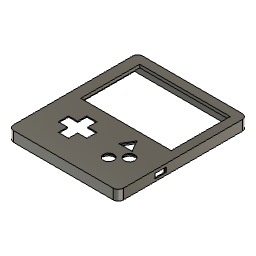
FINAL BMO Enclosure ECE 196 (Autodesk Fusion 360 design; units mm, degrees)
Autodesk Fusion 360 part; units mm, degrees
(part 1 of 2)
sketch "Sketch1" plane through (0, 0, 0) normal (0, 0, 1) x (1, 0, 0)
  line L0 (-50.4372, 47.8193) -> (49.5628, 47.8193)
  line L1 (49.5628, 47.8193) -> (49.5628, -63.1807)
  line L2 (49.5628, -63.1807) -> (-50.4372, -63.1807)
  line L3 (-50.4372, -63.1807) -> (-50.4372, 47.8193)
  line L4 (-18.6372, -27.5802) -> (-23.0372, -27.5802)
  line L5 (-23.0372, -27.5802) -> (-23.0372, -24.2802)
  line L6 (-23.0372, -24.2802) -> (-18.6372, -24.2802)
  line L7 (-18.6372, -24.2802) -> (-18.6372, -27.5802)
  line L8 (17.6628, -24.0807) -> (22.0628, -24.0807)
  line L9 (22.0628, -24.0807) -> (22.0628, -27.3807)
  line L10 (22.0628, -27.3807) -> (17.6628, -27.3807)
  line L11 (17.6628, -27.3807) -> (17.6628, -24.0807)
  line L12 (17.8378, -44.4057) -> (22.2378, -44.4057)
  line L13 (22.2378, -44.4057) -> (22.2378, -47.7057)
  line L14 (22.2378, -47.7057) -> (17.8378, -47.7057)
  line L15 (17.8378, -47.7057) -> (17.8378, -44.4057)
  line L16 (27.9628, -34.1807) -> (32.3628, -34.1807)
  line L17 (32.3628, -34.1807) -> (32.3628, -37.4807)
  line L18 (32.3628, -37.4807) -> (27.9628, -37.4807)
  line L19 (27.9628, -37.4807) -> (27.9628, -34.1807)
  line L20 (-33.0372, -34.1807) -> (-28.6372, -34.1807)
  line L21 (-28.6372, -34.1807) -> (-28.6372, -37.4807)
  line L22 (-28.6372, -37.4807) -> (-33.0372, -37.4807)
  line L23 (-33.0372, -37.4807) -> (-33.0372, -34.1807)
  line L24 (-13.0372, -34.1807) -> (-8.6372, -34.1807)
  line L25 (-8.6372, -34.1807) -> (-8.6372, -37.4807)
  line L26 (-8.6372, -37.4807) -> (-13.0372, -37.4807)
  line L27 (-13.0372, -37.4807) -> (-13.0372, -34.1807)
  line L28 (-23.4439, -44.4057) -> (-19.0439, -44.4057)
  line L29 (-19.0439, -44.4057) -> (-19.0439, -47.7057)
  line L30 (-19.0439, -47.7057) -> (-23.4439, -47.7057)
  line L31 (-23.4439, -47.7057) -> (-23.4439, -44.4057)
  dimension "d1" = 100
  dimension "d2" = 111
  dimension "d3" = 4.4
  dimension "d4" = 3.3
  dimension "d5" = 4.4
  dimension "d6" = 3.3
  dimension "d7" = 4.4
  dimension "d8" = 3.3
  dimension "d9" = 4.4
  dimension "d10" = 3.3
  dimension "d11" = 4.4
  dimension "d12" = 3.3
  dimension "d13" = 4.4
  dimension "d14" = 3.3
  dimension "d15" = 4.4
  dimension "d16" = 3.3
  dimension "d17" = 17.4
  dimension "d21" = 25.7
  dimension "d22" = 25.7
  dimension "d23" = 15.475
  dimension "d24" = 15.475
  dimension "d25" = 25.7
  dimension "d26" = 27.5
  dimension "d27" = 17.2
  dimension "d28" = 15.6
  dimension "d29" = 8.656
  dimension "d30" = 8.656
  dimension "d31" = 8.656
  dimension "d32" = 35.8
  dimension "d33" = 27.325
  constraint horizontal L0
  constraint vertical L1
  constraint horizontal L2
  constraint vertical L3
  constraint horizontal L4
  constraint vertical L5
  constraint horizontal L6
  constraint vertical L7
  constraint horizontal L8
  constraint vertical L9
  constraint horizontal L10
  constraint vertical L11
  constraint horizontal L12
  constraint vertical L13
  constraint horizontal L14
  constraint vertical L15
  constraint horizontal L16
  constraint vertical L17
  constraint horizontal L18
  constraint vertical L19
  constraint horizontal L20
  constraint vertical L21
  constraint horizontal L22
  constraint vertical L23
  constraint horizontal L24
  constraint vertical L25
  constraint horizontal L26
  constraint vertical L27
  constraint horizontal L28
  constraint vertical L29
  constraint horizontal L30
  constraint vertical L31
  measures "d1" distance of L0.start L0.end
  measures "d2" distance of L0.end L1.end
  measures "d3" distance of L4.start L4.end
  measures "d4" distance of L4.end L5.end
  measures "d5" distance of L28.start L28.end
  measures "d6" distance of L28.end L29.end
  measures "d7" distance of L24.start L24.end
  measures "d8" distance of L24.end L25.end
  measures "d9" distance of L20.start L20.end
  measures "d10" distance of L20.end L21.end
  measures "d11" distance of L8.start L8.end
  measures "d12" distance of L8.end L9.end
  measures "d13" distance of L16.start L16.end
  measures "d14" distance of L16.end L17.end
  measures "d15" distance of L12.start L12.end
  measures "d16" distance of L12.start L14.end
  measures "d17" distance of L3 L23
  measures "d21" distance of L2 L22
  measures "d22" distance of L2 L26
  measures "d23" distance of L2 L30
  measures "d24" distance of L2 L14
  measures "d25" distance of L2 L18
  measures "d26" distance of L1 L9
  measures "d27" distance of L1 L17
  measures "d28" distance of L21 L27
  measures "d29" distance of L4.end L20.end
  measures "d30" distance of L4.start L24.start
  measures "d31" distance of L21.end L28.start
  measures "d32" distance of L2 L10
  measures "d33" distance of L1 L13
sketch "top enclosure" plane through (0, 0, 0) normal (0, 0, 1) x (1, 0, 0)
  circle A0 centre (30.5628, -36.1807) radius 5.15
  line L0 (20.0628, -18.1807) -> (13.3583, -29.4363)
  line L1 (13.3583, -29.4363) -> (26.3583, -29.4363)
  line L2 (26.3583, -29.4363) -> (20.0628, -18.1807)
  circle A1 centre (20.0628, -46.1807) radius 5.15
  line L3 (-25.9372, -21.6807) -> (-15.9372, -21.6807)
  line L4 (-15.9372, -21.6807) -> (-15.9372, -30.6807)
  line L5 (-15.9372, -30.6807) -> (-6.9372, -30.6807)
  line L6 (-6.9372, -30.6807) -> (-6.9372, -40.6807)
  line L7 (-6.9372, -40.6807) -> (-15.9372, -40.6807)
  line L8 (-15.9372, -40.6807) -> (-15.9372, -49.6807)
  line L9 (-15.9372, -49.6807) -> (-25.9372, -49.6807)
  line L10 (-25.9372, -49.6807) -> (-25.9372, -40.6807)
  line L11 (-25.9372, -40.6807) -> (-34.9372, -40.6807)
  line L12 (-34.9372, -40.6807) -> (-34.9372, -30.6807)
  line L13 (-34.9372, -30.6807) -> (-25.9372, -30.6807)
  line L14 (-25.9372, -30.6807) -> (-25.9372, -21.6807)
  line L15 (-54.4372, 56.8193) -> (53.5628, 56.8193)
  line L16 (53.5628, 56.8193) -> (53.5628, -70.1807)
  line L17 (53.5628, -70.1807) -> (-54.4372, -70.1807)
  line L18 (-54.4372, -70.1807) -> (-54.4372, 56.8193)
  line L19 (-50.4372, -63.1807) -> (-50.4372, 47.8193)
  line L20 (49.5628, -63.1807) -> (-50.4372, -63.1807)
  line L21 (49.5628, 47.8193) -> (49.5628, -63.1807)
  line L22 (-50.4372, 47.8193) -> (49.5628, 47.8193)
  line L23 (-43.9372, 48.3193) -> (45.0628, 48.3193)
  line L24 (45.0628, 48.3193) -> (45.0628, -9.6807)
  line L25 (45.0628, -9.6807) -> (-43.9372, -9.6807)
  line L26 (-43.9372, -9.6807) -> (-43.9372, 48.3193)
  line L27 (-23.0372, -24.2802) -> (-18.6372, -24.2802)
  line L28 (-50.4372, -63.1807) -> (49.5628, -63.1807)
  line L29 (49.5628, -63.1807) -> (49.5628, 49.8193)
  line L30 (49.5628, 49.8193) -> (-50.4372, 49.8193)
  line L31 (-50.4372, 49.8193) -> (-50.4372, -63.1807)
  line L32 (44.9628, -13.6807) -> (49.5628, -13.6807)
  line L33 (49.5628, -13.6807) -> (49.5628, -23.1807)
  line L34 (49.5628, -23.1807) -> (44.9628, -23.1807)
  line L35 (44.9628, -23.1807) -> (44.9628, -13.6807)
  line L36 (-50.4372, -5.1807) -> (-36.8011, -5.1807)
  line L37 (-36.8011, -5.1807) -> (-36.8011, -27.1807)
  line L38 (-36.8011, -27.1807) -> (-50.4372, -27.1807)
  line L39 (-50.4372, -27.1807) -> (-50.4372, -5.1807)
  dimension "d34" = 60
  dimension "d35" = 10.3
  dimension "d36" = 10.3
  dimension "d37" = 10
  dimension "d38" = 10
  dimension "d39" = 10
  dimension "d40" = 10
  dimension "d41" = 9
  dimension "d42" = 9
  dimension "d43" = 9
  dimension "d44" = 9
  dimension "d45" = 9
  dimension "d46" = 9
  dimension "d47" = 13
  dimension "d49" = 11.2555
  dimension "d50" = 4
  dimension "d51" = 7
  dimension "d52" = 4
  dimension "d54" = 89
  dimension "d55" = 58
  dimension "d56" = 6.5
  dimension "d59" = 14.5995
  dimension "d60" = 45
  dimension "d61" = 27
  dimension "d62" = 17
  dimension "d63" = 13.5
  dimension "d64" = 15.5
  dimension "d65" = 19
  dimension "d66" = 29.5
  dimension "d68" = 113
  dimension "d69" = 100
  dimension "d72" = 40
  dimension "d73" = 9.5
  dimension "d74" = 4.6
  dimension "d75" = 36
  dimension "d77" = 22
  dimension "d230" = 7
  constraint horizontal L1
  constraint horizontal L3
  constraint perpendicular L3 L4
  constraint perpendicular L4 L5
  constraint perpendicular L5 L6
  constraint perpendicular L6 L7
  constraint perpendicular L7 L8
  constraint perpendicular L8 L9
  constraint perpendicular L9 L10
  constraint perpendicular L10 L11
  constraint perpendicular L11 L12
  constraint perpendicular L12 L13
  constraint perpendicular L3 L14
  constraint horizontal L15
  constraint vertical L16
  constraint horizontal L17
  constraint vertical L18
  constraint horizontal L23
  constraint vertical L24
  constraint horizontal L25
  constraint vertical L26
  constraint horizontal L28
  constraint vertical L29
  constraint horizontal L30
  constraint vertical L31
  constraint coincident L19.start L20.end
  constraint horizontal L32
  constraint vertical L33
  constraint horizontal L34
  constraint vertical L35
  constraint coincident L21 L33.end
  constraint horizontal L36
  constraint vertical L37
  constraint horizontal L38
  constraint vertical L39
  constraint coincident L19 L36.start
  measures "d34" angle of L0 L2
  measures "d35" diameter of A1
  measures "d36" diameter of A0
  measures "d37" distance of L3.start L3.end
  measures "d38" distance of L8.end L9.end
  measures "d39" distance of L5.end L6.end
  measures "d40" distance of L11.end L12.end
  measures "d41" distance of L3.start L13.end
  measures "d42" distance of L3.end L4.end
  measures "d43" distance of L4.end L5.end
  measures "d44" distance of L6.end L7.end
  measures "d45" distance of L9.end L10.end
  measures "d46" distance of L12.end L13.end
  measures "d47" distance of L0.end L1.end
  measures "d49" distance of L0.start L1
  measures "d50" distance of L18 L19
  measures "d51" distance of L17 L20
  measures "d52" distance of L16 L21
  measures "d54" distance of L23.start L23.end
  measures "d55" distance of L23.end L24.end
  measures "d56" distance of L19 L26
  measures "d59" distance of L25 L27
  measures "d60" distance of L0.start L20
  measures "d61" distance of A0.centre L20
  measures "d62" distance of A1.centre L20
  measures "d63" distance of L9 L20
  measures "d64" distance of L12 L19
  measures "d65" distance of A0.centre L21
  measures "d66" distance of L0.start L21
  measures "d68" distance of L19.start L30.end
  measures "d69" distance of L19.start L20.start
  measures "d72" distance of L20 L34
  measures "d73" distance of L32 L34
  measures "d74" distance of L33 L35
  measures "d75" distance of L28 L38
  measures "d77" distance of L36.end L37.end
  measures "d230" distance of L15 L30
extrude "Extrude6" add sketch "top enclosure" along normal blind 10 contours L15 L16 L17 L18 makes body 1
extrude "Extrude7" add sketch "top enclosure" along normal blind 3 contours L19 L20 L21 L22 L24 L25 L28 L29 L31 L32 L34 L35 L37 L38 | L19 L25 L26 L31 L36 L37 L38 L39 | L19 L22 L26 L31 L36 | L21 L29 L32 L33 L34 L35 | L22 L23 L24 L26 L29 L30 L31 bodies 1
sketch "Sketch3" plane through (53.5628, 0, 0) normal (1, 0, 0) x (0, 1, 0)
  line L0 (-70.1807, 0) -> (56.8193, 0)
  line L1 (56.8193, 0) -> (56.8193, 10)
  line L2 (56.8193, 10) -> (-70.1807, 10)
  line L3 (-70.1807, 10) -> (-70.1807, 0)
  line L4 (-34.1807, 7.5) -> (-23.1807, 7.5)
  line L5 (-23.1807, 7.5) -> (-23.1807, 3)
  line L6 (-23.1807, 3) -> (-34.1807, 3)
  line L7 (-34.1807, 3) -> (-34.1807, 7.5)
  line L8 (56.8193, 0) -> (-70.1807, 0)
  line L9 (-63.1807, 3) -> (-63.1807, 10)
  dimension "d92" = 3
  dimension "d93" = 11
  dimension "d94" = 4.5
  dimension "d212" = 40
  constraint horizontal L4
  constraint vertical L5
  constraint horizontal L6
  constraint vertical L7
  measures "d92" distance of L6 L8
  measures "d93" distance of L4.start L4.end
  measures "d94" distance of L4.end L5.end
  measures "d212" distance of L5 L9
extrude "Extrude8" cut sketch "Sketch3" against normal blind 10 contours L4 L5 L6 L7 bodies 1
sketch "Sketch4" plane through (49.5628, 0, 0) normal (-1, 0, 0) x (0, -1, 0)
  line L0 (23.1807, 3) -> (23.1807, 7.5)
  line L1 (23.1807, 7.5) -> (34.1807, 7.5)
  line L2 (34.1807, 7.5) -> (34.1807, 3)
  line L3 (34.1807, 3) -> (63.1807, 3)
  line L4 (63.1807, 3) -> (63.1807, 10)
  line L5 (63.1807, 10) -> (-49.8193, 10)
  line L6 (-49.8193, 10) -> (-49.8193, 3)
  line L7 (-49.8193, 3) -> (23.1807, 3)
  line L8 (21.9307, 3) -> (33.9307, 3)
  line L9 (33.9307, 3) -> (33.9307, 13)
  line L10 (33.9307, 13) -> (21.9307, 13)
  line L11 (21.9307, 13) -> (21.9307, 3)
  line L12 (23.1807, 7.5) -> (23.1807, 3)
  dimension "d97" = 12
  dimension "d98" = 10
  dimension "d99" = 1.25
  constraint horizontal L8
  constraint vertical L9
  constraint horizontal L10
  constraint vertical L11
  constraint coincident L7 L8.start
  measures "d97" distance of L9.end L10.end
  measures "d98" distance of L8.end L9.end
  measures "d99" distance of L11 L12
sketch "Sketch5" plane through (-54.4372, 0, 0) normal (-1, 0, 0) x (0, -1, 0)
  line L0 (-56.8193, 0) -> (70.1807, 0)
  line L1 (70.1807, 0) -> (70.1807, 10)
  line L2 (70.1807, 10) -> (-56.8193, 10)
  line L3 (-56.8193, 10) -> (-56.8193, 0)
  line L4 (8.1807, 7.5) -> (26.1807, 7.5)
  line L5 (26.1807, 7.5) -> (26.1807, 3)
  line L6 (26.1807, 3) -> (8.1807, 3)
  line L7 (8.1807, 3) -> (8.1807, 7.5)
  line L8 (63.1807, 3) -> (63.1807, 10)
  dimension "d103" = 18
  dimension "d104" = 3
  dimension "d105" = 4.5
  dimension "d174" = 55
  constraint horizontal L4
  constraint vertical L5
  constraint horizontal L6
  constraint vertical L7
  measures "d103" distance of L4.start L4.end
  measures "d104" distance of L0 L6
  measures "d105" distance of L4.end L5.end
  measures "d174" distance of L7 L8
sketch "Sketch6" plane through (-50.4372, 0, 0) normal (1, 0, 0) x (0, 1, 0)
  line L0 (49.8193, 3) -> (49.8193, 10)
  line L1 (49.8193, 10) -> (-63.1807, 10)
  line L2 (-63.1807, 10) -> (-63.1807, 3)
  line L3 (-63.1807, 3) -> (49.8193, 3)
  line L4 (-28.6807, 3) -> (-6.6807, 3)
  line L5 (-6.6807, 3) -> (-6.6807, 13)
  line L6 (-6.6807, 13) -> (-28.6807, 13)
  line L7 (-28.6807, 13) -> (-28.6807, 3)
  dimension "d111" = 22
  dimension "d112" = 10
  constraint horizontal L4
  constraint vertical L5
  constraint horizontal L6
  constraint vertical L7
  constraint coincident L3 L4.start
  measures "d111" distance of L5.end L6.end
  measures "d112" distance of L4.start L6.end
extrude "Extrude11" cut sketch "Sketch6" against normal blind 3 contours L1 L3 L4 L5 L7 | L1 L5 L6 L7 bodies 1
sketch "Sketch7" plane through (0, 0, 10) normal (0, 0, 1) x (-1, 0, 0)
  line L0 (50.4372, 28.6807) -> (53.4372, 28.6807)
  line L1 (53.4372, 28.6807) -> (53.4372, 6.6807)
  line L2 (53.4372, 6.6807) -> (50.4372, 6.6807)
  line L3 (50.4372, 6.6807) -> (50.4372, -49.8193)
  line L4 (50.4372, -49.8193) -> (-49.5628, -49.8193)
  line L5 (-49.5628, -49.8193) -> (-49.5628, 63.1807)
  line L6 (-49.5628, 63.1807) -> (50.4372, 63.1807)
  line L7 (50.4372, 63.1807) -> (50.4372, 28.6807)
  line L8 (54.4372, 70.1807) -> (-53.5628, 70.1807)
  line L9 (-53.5628, 70.1807) -> (-53.5628, -56.8193)
  line L10 (-53.5628, -56.8193) -> (54.4372, -56.8193)
  line L11 (54.4372, -56.8193) -> (54.4372, 70.1807)
  line L12 (54.4372, -56.8193) -> (-53.5628, -56.8193)
  line L13 (-53.5628, -56.8193) -> (-53.5628, 70.1807)
  line L14 (-53.5628, 70.1807) -> (54.4372, 70.1807)
  line L15 (54.4372, 70.1807) -> (54.4372, -56.8193)
  line L16 (50.4372, -49.8193) -> (-49.5628, -49.8193)
  line L17 (-49.5628, -49.8193) -> (-49.5628, 63.1807)
  line L18 (-49.5628, 63.1807) -> (50.4372, 63.1807)
  line L19 (50.4372, 63.1807) -> (50.4372, -49.8193)
  constraint horizontal L12
  constraint vertical L13
  constraint horizontal L14
  constraint vertical L15
  constraint coincident L8.end L9.start
  constraint coincident L10.end L11.start
  constraint horizontal L16
  constraint vertical L17
  constraint horizontal L18
  constraint vertical L19
  constraint coincident L5.end L6.start
  constraint coincident L3.end L4.start
extrude "Extrude12" add sketch "Sketch7" along normal blind 18.5 separate body contours L3 L4 L5 L6 L7 L16 L17 L18 L19 | L0 L1 L2 L19 | L8 L9 L10 L11 L12 L13 L14 L15 makes body 2
extrude "Extrude13" cut sketch "Sketch7" along normal blind 16 contours L3 L4 L5 L6 L7 L16 L17 L18 L19 bodies 2
sketch "Sketch9" plane through (53.5628, 0, 0) normal (1, 0, 0) x (0, 1, 0)
  line L0 (-70.1807, 10) -> (56.8193, 10)
  line L1 (56.8193, 10) -> (56.8193, 28.5)
  line L2 (56.8193, 28.5) -> (-70.1807, 28.5)
  line L3 (-70.1807, 28.5) -> (-70.1807, 10)
  line L4 (11.7578, 25.9206) -> (-35.8078, 25.9206) construction
  line L5 (-35.8078, 25.9206) -> (-35.8078, 11.4906) construction
  line L6 (-35.8078, 11.4906) -> (11.7578, 11.4906) construction
  line L7 (11.7578, 11.4906) -> (11.7578, 25.9206) construction
  dimension "d118" = 13
sketch "Sketch11" plane through (0, 0, 26) normal (0, 0, -1) x (1, 0, 0)
  line L0 (49.5628, 63.1807) -> (-50.4372, 63.1807)
  line L1 (-50.4372, 63.1807) -> (-50.4372, -49.8193)
  line L2 (-50.4372, -49.8193) -> (49.5628, -49.8193)
  line L3 (49.5628, -49.8193) -> (49.5628, 63.1807)
  line L4 (24.494, -23.0885) -> (41.494, -23.0885)
  line L5 (41.494, -23.0885) -> (41.494, 2.9115)
  line L6 (41.494, 2.9115) -> (24.494, 2.9115)
  line L7 (24.494, 2.9115) -> (24.494, -23.0885)
  ellipse E0 centre (32.994, -10.0885) end of major axis (32.994, 0) minor radius 7.0905
  line L8 (32.994, -20.177) -> (32.994, 0) construction
  line L9 (40.0845, -10.0885) -> (25.9034, -10.0885) construction
  dimension "d129" = 26
  dimension "d130" = 17
  constraint horizontal L4
  constraint vertical L5
  constraint horizontal L6
  constraint vertical L7
  constraint coincident E0 L8.start
  constraint coincident E0 L8.end
  constraint coincident E0 L9.start
  constraint coincident E0 L9.end
  constraint perpendicular L4 L8
  measures "d129" distance of L4.start L6.end
  measures "d130" distance of L5.end L6.end
sketch "Sketch12" plane through (0, 0, 3) normal (0, 0, 1) x (-1, 0, 0)
  line L0 (50.4372, 28.6807) -> (50.4372, 63.1807)
  line L1 (50.4372, 63.1807) -> (-49.5628, 63.1807)
  line L2 (-49.5628, 63.1807) -> (-49.5628, 34.1807)
  line L3 (-49.5628, 34.1807) -> (-53.5628, 34.1807)
  line L4 (-53.5628, 34.1807) -> (-53.5628, 23.1807)
  line L5 (-53.5628, 23.1807) -> (-49.5628, 23.1807)
  line L6 (-49.5628, 23.1807) -> (-49.5628, -49.8193)
  line L7 (-49.5628, -49.8193) -> (50.4372, -49.8193)
  line L8 (50.4372, -49.8193) -> (50.4372, 6.6807)
  line L9 (50.4372, 6.6807) -> (53.4372, 6.6807)
  line L10 (53.4372, 6.6807) -> (53.4372, 28.6807)
  line L11 (-45.0628, -48.3193) -> (-45.0628, 9.6807)
  line L12 (-45.0628, 9.6807) -> (43.9372, 9.6807)
  line L13 (43.9372, 9.6807) -> (43.9372, -48.3193)
  line L14 (43.9372, -48.3193) -> (-45.0628, -48.3193)
  circle A0 centre (-30.5628, 36.1807) radius 5.15
  line L15 (-20.0628, 18.1807) -> (-26.3583, 29.4363)
  line L16 (-26.3583, 29.4363) -> (-13.3583, 29.4363)
  line L17 (-13.3583, 29.4363) -> (-20.0628, 18.1807)
  circle A1 centre (-20.0628, 46.1807) radius 5.15
  line L18 (34.9372, 30.6807) -> (25.9372, 30.6807)
  line L19 (25.9372, 30.6807) -> (25.9372, 21.6807)
  line L20 (25.9372, 21.6807) -> (15.9372, 21.6807)
  line L21 (15.9372, 21.6807) -> (15.9372, 30.6807)
  line L22 (15.9372, 30.6807) -> (6.9372, 30.6807)
  line L23 (6.9372, 30.6807) -> (6.9372, 40.6807)
  line L24 (6.9372, 40.6807) -> (15.9372, 40.6807)
  line L25 (15.9372, 40.6807) -> (15.9372, 49.6807)
  line L26 (15.9372, 49.6807) -> (25.9372, 49.6807)
  line L27 (25.9372, 49.6807) -> (25.9372, 40.6807)
  line L28 (25.9372, 40.6807) -> (34.9372, 40.6807)
  line L29 (34.9372, 40.6807) -> (34.9372, 30.6807)
  line L30 (15.9372, 30.6807) -> (6.9372, 30.6807)
  line L31 (6.9372, 30.6807) -> (6.9372, 40.6807)
  line L32 (15.9372, 40.6807) -> (15.9372, 49.6807)
  line L33 (15.9372, 49.6807) -> (25.9372, 49.6807)
  line L34 (25.9372, 49.6807) -> (25.9372, 40.6807)
  line L35 (34.9372, 40.6807) -> (34.9372, 30.6807)
  line L36 (34.9372, 30.6807) -> (25.9372, 30.6807)
  line L37 (25.9372, 21.6807) -> (15.9372, 21.6807)
  line L38 (15.9372, 21.6807) -> (15.9372, 30.6807)
  line L39 (25.9372, 30.6807) -> (25.9372, 21.6807)
  line L40 (-28.0634, 30.4363) -> (-11.5986, 30.4363)
  line L41 (-11.5986, 30.4363) -> (-20.0901, 16.1809)
  line L42 (-20.0901, 16.1809) -> (-28.0634, 30.4363)
  circle A2 centre (-30.5628, 36.1807) radius 6.15
  circle A3 centre (-20.0628, 46.1807) radius 6.15
  line L43 (4.9372, 28.6807) -> (4.9372, 42.6807)
  line L44 (4.9372, 42.6807) -> (13.9372, 42.6807)
  line L45 (13.9372, 42.6807) -> (13.9372, 51.6807)
  line L46 (13.9372, 51.6807) -> (27.9372, 51.6807)
  line L47 (27.9372, 51.6807) -> (27.9372, 42.6807)
  line L48 (27.9372, 42.6807) -> (36.9372, 42.6807)
  line L49 (36.9372, 42.6807) -> (36.9372, 28.6807)
  line L50 (36.9372, 28.6807) -> (27.9372, 28.6807)
  line L51 (27.9372, 28.6807) -> (27.9372, 19.6807)
  line L52 (27.9372, 19.6807) -> (13.9372, 19.6807)
  line L53 (13.9372, 19.6807) -> (13.9372, 28.6807)
  line L54 (13.9372, 28.6807) -> (4.9372, 28.6807)
  line L55 (53.4372, 28.6807) -> (50.4372, 28.6807)
  line L56 (-13.965, 45.3815) -> (-10, 45.3815)
  line L57 (-10, 45.3815) -> (-10, 48)
  line L58 (-10, 48) -> (-14.188, 48)
  line L59 (-36.6796, 36.8191) -> (-40.3994, 36.8191)
  line L60 (-40.3994, 36.8191) -> (-40.3994, 34)
  line L61 (-40.3994, 34) -> (-36.3132, 34)
  line L62 (-13.965, 45.3815) -> (-14.188, 48)
  line L63 (-36.3132, 34) -> (-36.6796, 36.8191)
  dimension "d145" = -1
  dimension "d146" = 1
  dimension "d147" = 1
  dimension "d148" = -2
  constraint coincident A3 L56.start
  constraint horizontal L56
  constraint perpendicular L56 L57
  constraint coincident A3 L58.end
  constraint perpendicular L57 L58
  constraint coincident A2 L59.start
  constraint parallel L12 L59
  constraint perpendicular L12 L60
  constraint coincident A2 L61.end
  constraint perpendicular L60 L61
extrude "Extrude20" cut sketch "Sketch12" against normal blind 2 contours L43 L44 L45 L46 L47 L48 L49 L50 L51 L52 L53 L54 bodies 1
extrude "Extrude21" cut sketch "Sketch12" against normal blind 2 contours L40 L41 L42 | A2 L63 | A2 L63 | A2 L59 L60 L61 | A3 L62 | A3 L56 L57 L58 | A3 L62 bodies 1
sketch "Sketch13" plane through (49.5628, 0, 0) normal (-1, 0, 0) x (0, -1, 0)
  line L0 (23.1807, 3) -> (23.1807, 7.5)
  line L1 (23.1807, 7.5) -> (34.1807, 7.5)
  line L2 (34.1807, 7.5) -> (34.1807, 3)
  line L3 (34.1807, 3) -> (63.1807, 3)
  line L4 (63.1807, 3) -> (63.1807, 10)
  line L5 (63.1807, 10) -> (-49.8193, 10)
  line L6 (-49.8193, 10) -> (-49.8193, 3)
  line L7 (-49.8193, 3) -> (23.1807, 3)
  line L8 (21.1807, 3) -> (36.1807, 3)
  line L9 (36.1807, 3) -> (36.1807, 11.5)
  line L10 (36.1807, 11.5) -> (21.1807, 11.5)
  line L11 (21.1807, 11.5) -> (21.1807, 3)
  dimension "d154" = 2
  dimension "d155" = 2
  dimension "d156" = 4
  constraint horizontal L8
  constraint vertical L9
  constraint horizontal L10
  constraint vertical L11
  constraint coincident L7 L8.start
  measures "d154" distance of L0 L11
  measures "d155" distance of L2 L9
  measures "d156" distance of L1 L10
extrude "Extrude22" cut sketch "Sketch13" against normal blind 3 contours L0 L1 L2 L3 L5 L7 L8 L9 L11 bodies 1
fillet "Fillet1" radius 5 1 edges at (-54.4372, 56.8193, 19.25) on bodies 2
fillet "Fillet2" radius 5 1 edges at (-54.4372, 56.8193, 5) on bodies 1
fillet "Fillet3" radius 5 2 edges at (-54.4372, -70.1807, 5) (-54.4372, -70.1807, 19.25) on bodies 1 2
fillet "Fillet4" radius 5 2 edges at (53.5628, 56.8193, 5) (53.5628, 56.8193, 19.25) on bodies 1 2
fillet "Fillet5" radius 5 2 edges at (53.5628, -70.1807, 5) (53.5628, -70.1807, 19.25) on bodies 1 2
sketch "Sketch14" plane through (0, 0, 1) normal (0, 0, 1) x (-1, 0, 0)
  line L0 (34.9372, 30.6807) -> (25.9372, 30.6807)
  line L1 (25.9372, 30.6807) -> (25.9372, 21.6807)
  line L2 (25.9372, 21.6807) -> (15.9372, 21.6807)
  line L3 (15.9372, 21.6807) -> (15.9372, 30.6807)
  line L4 (15.9372, 30.6807) -> (6.9372, 30.6807)
  line L5 (6.9372, 30.6807) -> (6.9372, 40.6807)
  line L6 (6.9372, 40.6807) -> (15.9372, 40.6807)
  line L7 (15.9372, 40.6807) -> (15.9372, 49.6807)
  line L8 (15.9372, 49.6807) -> (25.9372, 49.6807)
  line L9 (25.9372, 49.6807) -> (25.9372, 40.6807)
  line L10 (25.9372, 40.6807) -> (34.9372, 40.6807)
  line L11 (34.9372, 40.6807) -> (34.9372, 30.6807)
  line L12 (13.9372, 28.6807) -> (13.9372, 19.6807)
  line L13 (13.9372, 19.6807) -> (27.9372, 19.6807)
  line L14 (27.9372, 19.6807) -> (27.9372, 28.6807)
  line L15 (27.9372, 28.6807) -> (36.9372, 28.6807)
  line L16 (36.9372, 28.6807) -> (36.9372, 42.6807)
  line L17 (36.9372, 42.6807) -> (27.9372, 42.6807)
  line L18 (27.9372, 42.6807) -> (27.9372, 51.6807)
  line L19 (27.9372, 51.6807) -> (13.9372, 51.6807)
  line L20 (13.9372, 51.6807) -> (13.9372, 42.6807)
  line L21 (13.9372, 42.6807) -> (4.9372, 42.6807)
  line L22 (4.9372, 42.6807) -> (4.9372, 28.6807)
  line L23 (4.9372, 28.6807) -> (13.9372, 28.6807)
  line L24 (14.7372, 20.4807) -> (27.1372, 20.4807)
  line L25 (27.1372, 20.4807) -> (27.1372, 29.4807)
  line L26 (27.1372, 29.4807) -> (36.1372, 29.4807)
  line L27 (36.1372, 29.4807) -> (36.1372, 41.8807)
  line L28 (36.1372, 41.8807) -> (27.1372, 41.8807)
  line L29 (27.1372, 41.8807) -> (27.1372, 50.8807)
  line L30 (27.1372, 50.8807) -> (14.7372, 50.8807)
  line L31 (14.7372, 50.8807) -> (14.7372, 41.8807)
  line L32 (14.7372, 41.8807) -> (5.7372, 41.8807)
  line L33 (5.7372, 41.8807) -> (5.7372, 29.4807)
  line L34 (5.7372, 29.4807) -> (14.7372, 29.4807)
  line L35 (14.7372, 29.4807) -> (14.7372, 20.4807)
  dimension "d175" = -0.8
sketch "Sketch15" plane through (0, 0, 1) normal (0, 0, 1) x (-1, 0, 0)
  line L0 (-26.3583, 29.4363) -> (-13.3583, 29.4363)
  line L1 (-13.3583, 29.4363) -> (-20.0628, 18.1807)
  line L2 (-20.0628, 18.1807) -> (-26.3583, 29.4363)
  line L3 (-20.0901, 16.1809) -> (-11.5986, 30.4363)
  line L4 (-11.5986, 30.4363) -> (-28.0634, 30.4363)
  line L5 (-28.0634, 30.4363) -> (-20.0901, 16.1809)
  line L6 (-12.3025, 30.0363) -> (-27.3813, 30.0363)
  line L7 (-27.3813, 30.0363) -> (-20.0791, 16.9808)
  line L8 (-20.0791, 16.9808) -> (-12.3025, 30.0363)
  dimension "d176" = -0.4
sketch "Sketch16" plane through (0, 0, 1) normal (0, 0, 1) x (-1, 0, 0)
  circle A0 centre (-30.5628, 36.1807) radius 5.15
  circle A1 centre (-30.5628, 36.1807) radius 5.75
  line L0 (-40.3994, 34) -> (-36.3132, 34)
  arc A2 (-36.3132, 34) -> (-36.6796, 36.8191) centre (-30.5628, 36.1807) ccw
  line L1 (-36.6796, 36.8191) -> (-40.3994, 36.8191)
  line L2 (-40.3994, 36.8191) -> (-40.3994, 34)
  line L3 (-36.0013, 34.3137) -> (-40, 34.3137)
  line L4 (-40, 34.3137) -> (-40, 36.5)
  line L5 (-40, 36.5) -> (-36.3039, 36.5)
  constraint coincident A1 L3.start
  constraint horizontal L3
  constraint perpendicular L3 L4
  constraint coincident A1 L5.end
  constraint perpendicular L4 L5
sketch "Sketch17" plane through (0, 0, 1) normal (0, 0, 1) x (-1, 0, 0)
  circle A0 centre (-20.0628, 46.1807) radius 5.15
  circle A1 centre (-20.0628, 46.1807) radius 5.75
  line L0 (-10, 48) -> (-14.188, 48)
  arc A2 (-14.188, 48) -> (-13.965, 45.3815) centre (-20.0628, 46.1807) ccw
  line L1 (-13.965, 45.3815) -> (-10, 45.3815)
  line L2 (-10, 45.3815) -> (-10, 48)
  line L3 (-14.332, 45.7107) -> (-10.2595, 45.7107)
  line L4 (-10.2595, 45.7107) -> (-10.2595, 47.6884)
  line L5 (-10.2595, 47.6884) -> (-14.514, 47.6884)
  constraint coincident A1 L3.start
  constraint parallel L1 L3
  constraint perpendicular L3 L4
  constraint coincident A1 L5.end
  constraint perpendicular L4 L5
extrude "Extrude23" add sketch "Sketch14" sketch "Sketch15" sketch "Sketch16" sketch "Sketch17" along normal up to surface separate body contours L0 L1 L2 L3 L4 L5 L6 L7 L8 L9 L10 L11 | L24 L25 L26 L27 L28 L29 L30 L31 L32 L33 L34 L35 of sketch 2 contours L0 L1 L2 | L6 L7 L8 of sketch 3 contours A0 | A1 | A1 L3 L4 L5 of sketch 4 contours A0 | A1 | A1 L3 L4 L5 end surface through (0, 0, 10) normal (0, 0, 1) offset -4.6 makes body 3 at (35.053, -32.589, 3.9333) makes body 4 at (19.921, -25.6845, 1) makes body 5 at (-23.0039, -37.7474, 1) makes body 6 at (24.8522, -42.9988, 3.9333)
sketch "Sketch22" plane through (0, 0, 1) normal (0, 0, -1) x (1, 0, 0)
  line L0 (12.3025, 30.0363) -> (20.0791, 16.9808)
  line L1 (20.0791, 16.9808) -> (27.3813, 30.0363)
  line L2 (27.3813, 30.0363) -> (12.3025, 30.0363)
  line L3 (26.0172, 29.2363) -> (13.7102, 29.2363)
  line L4 (13.7102, 29.2363) -> (20.0573, 18.5807)
  line L5 (20.0573, 18.5807) -> (26.0172, 29.2363)
  dimension "d187" = -0.8
sketch "Sketch23" plane through (0, 0, 1) normal (0, 0, -1) x (1, 0, 0)
  circle A0 centre (30.5628, 36.1807) radius 4.85
  arc A1 (36.3039, 36.5) -> (36.0013, 34.3137) centre (30.5628, 36.1807) ccw
  line L0 (36.0013, 34.3137) -> (40, 34.3137)
  line L1 (40, 34.3137) -> (40, 36.5)
  line L2 (40, 36.5) -> (36.3039, 36.5)
  line L3 (12.3025, 30.0363) -> (20.0791, 16.9808)
  line L4 (20.0791, 16.9808) -> (27.3813, 30.0363)
  line L5 (27.3813, 30.0363) -> (12.3025, 30.0363)
  line L6 (14.514, 47.6884) -> (10.2595, 47.6884)
  line L7 (10.2595, 47.6884) -> (10.2595, 45.7107)
  line L8 (10.2595, 45.7107) -> (14.332, 45.7107)
  arc A2 (14.332, 45.7107) -> (14.514, 47.6884) centre (20.0628, 46.1807) ccw
  line L9 (-14.7372, 20.4807) -> (-14.7372, 29.4807)
  line L10 (-14.7372, 29.4807) -> (-5.7372, 29.4807)
  line L11 (-5.7372, 29.4807) -> (-5.7372, 41.8807)
  line L12 (-5.7372, 41.8807) -> (-14.7372, 41.8807)
  line L13 (-14.7372, 41.8807) -> (-14.7372, 50.8807)
  line L14 (-14.7372, 50.8807) -> (-27.1372, 50.8807)
  line L15 (-27.1372, 50.8807) -> (-27.1372, 41.8807)
  line L16 (-27.1372, 41.8807) -> (-36.1372, 41.8807)
  line L17 (-36.1372, 41.8807) -> (-36.1372, 29.4807)
  line L18 (-36.1372, 29.4807) -> (-27.1372, 29.4807)
  line L19 (-27.1372, 29.4807) -> (-27.1372, 20.4807)
  line L20 (-27.1372, 20.4807) -> (-14.7372, 20.4807)
  constraint concentric A0 A1
sketch "Sketch24" plane through (0, 0, 1) normal (0, 0, -1) x (1, 0, 0)
  line L0 (-14.7372, 20.4807) -> (-14.7372, 29.4807)
  line L1 (-14.7372, 29.4807) -> (-5.7372, 29.4807)
  line L2 (-5.7372, 29.4807) -> (-5.7372, 41.8807)
  line L3 (-5.7372, 41.8807) -> (-14.7372, 41.8807)
  line L4 (-14.7372, 41.8807) -> (-14.7372, 50.8807)
  line L5 (-14.7372, 50.8807) -> (-27.1372, 50.8807)
  line L6 (-27.1372, 50.8807) -> (-27.1372, 41.8807)
  line L7 (-27.1372, 41.8807) -> (-36.1372, 41.8807)
  line L8 (-36.1372, 41.8807) -> (-36.1372, 29.4807)
  line L9 (-36.1372, 29.4807) -> (-27.1372, 29.4807)
  line L10 (-27.1372, 29.4807) -> (-27.1372, 20.4807)
  line L11 (-27.1372, 20.4807) -> (-14.7372, 20.4807)
  line L12 (-16.2372, 30.9807) -> (-7.2372, 30.9807)
  line L13 (-7.2372, 30.9807) -> (-7.2372, 40.3807)
  line L14 (-7.2372, 40.3807) -> (-16.2372, 40.3807)
  line L15 (-16.2372, 40.3807) -> (-16.2372, 49.3807)
  line L16 (-16.2372, 49.3807) -> (-25.6372, 49.3807)
  line L17 (-25.6372, 49.3807) -> (-25.6372, 40.3807)
  line L18 (-25.6372, 40.3807) -> (-34.6372, 40.3807)
  line L19 (-34.6372, 40.3807) -> (-34.6372, 30.9807)
  line L20 (-34.6372, 30.9807) -> (-25.6372, 30.9807)
  line L21 (-25.6372, 30.9807) -> (-25.6372, 21.9807)
  line L22 (-25.6372, 21.9807) -> (-16.2372, 21.9807)
  line L23 (-16.2372, 21.9807) -> (-16.2372, 30.9807)
  dimension "d189" = -1.5
sketch "Sketch25" plane through (0, 0, 1) normal (0, 0, -1) x (1, 0, 0)
  circle A0 centre (30.5628, 36.1807) radius 4.85
  arc A1 (36.3039, 36.5) -> (36.0013, 34.3137) centre (30.5628, 36.1807) ccw
  line L0 (36.0013, 34.3137) -> (40, 34.3137)
  line L1 (40, 34.3137) -> (40, 36.5)
  line L2 (40, 36.5) -> (36.3039, 36.5)
  line L3 (12.3025, 30.0363) -> (20.0791, 16.9808)
  line L4 (20.0791, 16.9808) -> (27.3813, 30.0363)
  line L5 (27.3813, 30.0363) -> (12.3025, 30.0363)
  line L6 (14.514, 47.6884) -> (10.2595, 47.6884)
  line L7 (10.2595, 47.6884) -> (10.2595, 45.7107)
  line L8 (10.2595, 45.7107) -> (14.332, 45.7107)
  arc A2 (14.332, 45.7107) -> (14.514, 47.6884) centre (20.0628, 46.1807) ccw
  line L9 (-14.7372, 20.4807) -> (-14.7372, 29.4807)
  line L10 (-14.7372, 29.4807) -> (-5.7372, 29.4807)
  line L11 (-5.7372, 29.4807) -> (-5.7372, 41.8807)
  line L12 (-5.7372, 41.8807) -> (-14.7372, 41.8807)
  line L13 (-14.7372, 41.8807) -> (-14.7372, 50.8807)
  line L14 (-14.7372, 50.8807) -> (-27.1372, 50.8807)
  line L15 (-27.1372, 50.8807) -> (-27.1372, 41.8807)
  line L16 (-27.1372, 41.8807) -> (-36.1372, 41.8807)
  line L17 (-36.1372, 41.8807) -> (-36.1372, 29.4807)
  line L18 (-36.1372, 29.4807) -> (-27.1372, 29.4807)
  line L19 (-27.1372, 29.4807) -> (-27.1372, 20.4807)
  line L20 (-27.1372, 20.4807) -> (-14.7372, 20.4807)
  circle A3 centre (20.0628, 46.1807) radius 5.1598
  circle A4 centre (20.0628, 46.1807) radius 4.8598
  dimension "d207" = -0.3
  constraint concentric A0 A1
  constraint concentric A2 A3
extrude "Extrude25" add sketch "Sketch23" sketch "Sketch22" sketch "Sketch25" sketch "Sketch24" along normal blind 2.5 contours A0 of sketch 2 contours L3 L4 L5 of sketch 3 contours A0 of sketch 4 contours L12 L13 L14 L15 L16 L17 L18 L19 L20 L21 L22 L23 bodies 3 5 4
sketch "Sketch26" plane through (0, 0, -1.5) normal (0, 0, -1) x (1, 0, 0)
  line L0 (-16.2372, 21.9807) -> (-16.2372, 30.9807)
  line L1 (-16.2372, 30.9807) -> (-7.2372, 30.9807)
  line L2 (-7.2372, 30.9807) -> (-7.2372, 40.3807)
  line L3 (-7.2372, 40.3807) -> (-16.2372, 40.3807)
  line L4 (-16.2372, 40.3807) -> (-16.2372, 49.3807)
  line L5 (-16.2372, 49.3807) -> (-25.6372, 49.3807)
  line L6 (-25.6372, 49.3807) -> (-25.6372, 40.3807)
  line L7 (-25.6372, 40.3807) -> (-34.6372, 40.3807)
  line L8 (-34.6372, 40.3807) -> (-34.6372, 30.9807)
  line L9 (-34.6372, 30.9807) -> (-25.6372, 30.9807)
  line L10 (-25.6372, 30.9807) -> (-25.6372, 21.9807)
  line L11 (-25.6372, 21.9807) -> (-16.2372, 21.9807)
  circle A0 centre (-20.9372, 35.6807) radius 3
  dimension "d193" = 6
  measures "d193" diameter of A0
extrude "Extrude26" cut sketch "Sketch26" against normal blind 0.3 contours A0 bodies 5
fillet "Fillet6" radius 0.3 1 edges at (-23.7342, -36.7656, -1.5) on bodies 5
sketch "Sketch27" plane through (0, 0, -1.5) normal (0, 0, -1) x (1, 0, 0)
  line L0 (20.0573, 18.5807) -> (26.0172, 29.2363)
  line L1 (26.0172, 29.2363) -> (13.7102, 29.2363)
  line L2 (13.7102, 29.2363) -> (20.0573, 18.5807)
  line L3 (21, 28) -> (19, 28) construction
  line L4 (19, 28) -> (19, 23) construction
  line L5 (19, 23) -> (21, 23) construction
  line L6 (21, 23) -> (21, 28) construction
  line L7 (32.948, 39.073) -> (28.0236, 39.0916) construction
  line L8 (28.0236, 39.0916) -> (28.0006, 33.0191) construction
  line L9 (28.0006, 33.0191) -> (32.925, 33.0005) construction
  line L10 (32.925, 33.0005) -> (32.948, 39.073) construction
  line L11 (22.1916, 49.0811) -> (17.5135, 49.0529) construction
  line L12 (17.5135, 49.0529) -> (17.5465, 43.5713) construction
  line L13 (17.5465, 43.5713) -> (22.2246, 43.5995) construction
  line L14 (22.2246, 43.5995) -> (22.1916, 49.0811) construction
  dimension "d198" = 5
  dimension "d199" = 5
  dimension "d200" = 5
  text T0 "S" font "Arial" height 5 align centre middle in box 2 x 5 at (21, 28) x (-1, 0) y (0, -1) spacing 1 kerned
  text T1 "D" font "Arial" height 5 align centre middle in box 4.9245 x 6.0725 at (32.948, 39.073) x (-0.999993, 0.003785) y (-0.003785, -0.999993) spacing 1 kerned
  text T2 "B" font "Arial" height 5 align centre middle in box 4.6781 x 5.4817 at (22.1916, 49.0811) x (-0.999982, -0.006022) y (0.006022, -0.999982) spacing 1 kerned
extrude "Extrude28" cut sketch "Sketch27" against normal blind 0.5 text T1 T2 T0 bodies 3 4
extrude "Extrude29" cut sketch "Sketch27" against normal blind 0.6 text T0 bodies 4
extrude "Extrude30" add sketch "Sketch25" along normal blind 2.5 contours A4 bodies 6
extrude "Extrude31" cut sketch "Sketch27" against normal blind 0.5 text T2 bodies 6
sketch "Sketch29" plane through (-54.4372, 0, 0) normal (-1, 0, 0) x (0, -1, 0)
  line L0 (28.6079, 8.2636) -> (6.6079, 8.2636)
  line L1 (6.6079, 8.2636) -> (6.6079, 14.2636)
  line L2 (6.6079, 14.2636) -> (28.6079, 14.2636)
  line L3 (28.6079, 14.2636) -> (28.6079, 8.2636)
  dimension "d213" = 6
  dimension "d214" = 22
  constraint horizontal L0
  constraint vertical L1
  constraint horizontal L2
  constraint vertical L3
  measures "d213" distance of L0.start L2.end
  measures "d214" distance of L0.start L0.end
extrude "Extrude32" cut sketch "Sketch29" against normal blind 6 bodies 1 2
sketch "Sketch30" plane through (49.5628, 0, 0) normal (-1, 0, 0) x (0, -1, 0)
  line L0 (-49.8193, 10) -> (63.1807, 10)
  line L1 (63.1807, 10) -> (63.1807, 26)
  line L2 (63.1807, 26) -> (-49.8193, 26)
  line L3 (-49.8193, 26) -> (-49.8193, 10)
  line L4 (-23.7308, 10.6685) -> (-38.7308, 10.6685)
  line L5 (-23.8198, 25.7685) -> (-38.8198, 25.7685)
  arc A0 (-23.7308, 10.6685) -> (-23.8198, 25.7685) centre (-25.1353, 18.2105) ccw
  arc A1 (-38.8198, 25.7685) -> (-38.7308, 10.6685) centre (-37.6054, 18.2254) ccw
  circle A2 centre (-31.599, 12.6391) radius 1.25
  circle A3 centre (-31.4598, 17.937) radius 1.25
  circle A4 centre (-26.9413, 15.1675) radius 1.25
  circle A5 centre (-26.8021, 20.4654) radius 1.25
  circle A6 centre (-31.3206, 23.235) radius 1.25
  circle A7 centre (-35.9784, 20.7066) radius 1.25
  circle A8 centre (-36.1176, 15.4086) radius 1.25
  dimension "d217" = 15.1
  dimension "d218" = 15
  dimension "d219" = 15
  dimension "d220" = 7.6717
  dimension "d221" = 7.6402
  dimension "d224" = 2.5
  dimension "d225" = 2.5
  dimension "d227" = 360
  constraint horizontal L4
  constraint parallel L2 L5
  measures "d217" distance of L4 L5
  measures "d218" distance of L4.start L4.end
  measures "d219" distance of L5.start L5.end
  measures "d220" radius of A0
  measures "d221" radius of A1
  measures "d224" diameter of A2
  measures "d225" diameter of A3
extrude "Extrude33" cut sketch "Sketch30" against normal blind 3.3 contours L4 L5 A0 A1 | A2 | A3 | A4 | A5 | A6 | A7 | A8 bodies 2
extrude "Extrude34" cut sketch "Sketch30" against normal blind 5 contours A2 | A3 | A4 | A5 | A6 | A7 | A8 bodies 2
sketch "Sketch31" plane through (0, 0, 10) normal (0, 0, -1) x (1, 0, 0)
  line L0 (-50.4372, 6.6079) -> (-54.4372, 6.6079)
  line L1 (-54.4372, 6.6079) -> (-54.4372, -51.8193)
  arc A0 (-54.4372, -51.8193) -> (-49.4372, -56.8193) centre (-49.4372, -51.8193) ccw
  line L2 (-49.4372, -56.8193) -> (48.5628, -56.8193)
  arc A1 (48.5628, -56.8193) -> (53.5628, -51.8193) centre (48.5628, -51.8193) ccw
  line L3 (53.5628, -51.8193) -> (53.5628, 65.1807)
  arc A2 (53.5628, 65.1807) -> (48.5628, 70.1807) centre (48.5628, 65.1807) ccw
  line L4 (48.5628, 70.1807) -> (-49.4372, 70.1807)
  arc A3 (-49.4372, 70.1807) -> (-54.4372, 65.1807) centre (-49.4372, 65.1807) ccw
  line L5 (-54.4372, 65.1807) -> (-54.4372, 28.6079)
  line L6 (-54.4372, 28.6079) -> (-50.4372, 28.6079)
  line L7 (-50.4372, 28.6079) -> (-50.4372, 63.1807)
  line L8 (-50.4372, 63.1807) -> (49.5628, 63.1807)
  line L9 (49.5628, 63.1807) -> (49.5628, -49.8193)
  line L10 (49.5628, -49.8193) -> (-50.4372, -49.8193)
  line L11 (-50.4372, -49.8193) -> (-50.4372, 6.6079)
  circle A4 centre (-36.2346, 66.4664) radius 2.725
  circle A5 centre (37.4116, 66.6526) radius 2.725
  circle A6 centre (-36.7046, -53.3293) radius 2.725
  circle A7 centre (35.1958, -53.3905) radius 2.725
  circle A8 centre (-36.2346, 66.4664) radius 1.5
  circle A9 centre (37.4116, 66.6526) radius 1.5
  circle A10 centre (-36.7046, -53.3293) radius 1.5
  circle A11 centre (35.1958, -53.3905) radius 1.5
  dimension "d231" = 5.45
  dimension "d232" = 5.45
  dimension "d233" = 5.45
  dimension "d234" = 5.45
  dimension "d235" = 3
  dimension "d236" = 3
  dimension "d237" = 3
  dimension "d238" = 3
  constraint concentric A4 A8
  constraint concentric A5 A9
  constraint concentric A6 A10
  constraint concentric A7 A11
  measures "d231" diameter of A4
  measures "d232" diameter of A5
  measures "d233" diameter of A6
  measures "d234" diameter of A7
  measures "d235" diameter of A8
  measures "d236" diameter of A9
  measures "d237" diameter of A10
  measures "d238" diameter of A11
extrude "Extrude35" cut sketch "Sketch31" along normal blind 4.5 and the other way blind 7 contours A8 | A9 | A10 | A11 bodies 1 2
extrude "Extrude36" cut sketch "Sketch31" against normal blind 16 from surface at -7 contours A4 | A5 | A6 | A7 | A8 | A9 | A10 | A11 bodies 2
sketch "Sketch32" plane through (-54.4372, 0, 0) normal (-1, 0, 0) x (0, -1, 0)
  line L0 (6.6079, 10) -> (6.6079, 14.2636)
  line L1 (6.6079, 14.2636) -> (28.6079, 14.2636)
  line L2 (28.6079, 14.2636) -> (28.6079, 10)
  line L3 (28.6079, 10) -> (65.1807, 10)
  line L4 (65.1807, 10) -> (65.1807, 28.5)
  line L5 (65.1807, 28.5) -> (-51.8193, 28.5)
  line L6 (-51.8193, 28.5) -> (-51.8193, 10)
  line L7 (-51.8193, 10) -> (6.6079, 10)
  line L8 (-39.1193, 16.5) -> (-12.1193, 16.5)
  line L9 (-12.1193, 16.5) -> (-12.1193, 10)
  line L10 (-12.1193, 10) -> (-39.1193, 10)
  line L11 (-39.1193, 10) -> (-39.1193, 16.5)
  line L12 (-56.8193, 28.5) -> (-56.8193, 10)
  dimension "d246" = 17.7
  dimension "d247" = 27
  dimension "d248" = 6.5
  constraint horizontal L8
  constraint vertical L9
  constraint horizontal L10
  constraint vertical L11
  constraint coincident L7 L9.end
  measures "d246" distance of L11 L12
  measures "d247" distance of L8.start L8.end
  measures "d248" distance of L8.end L9.end
extrude "Extrude37" cut sketch "Sketch32" against normal blind 5 contours L7 L8 L9 L10 L11 bodies 2
ref_plane "WorkPlane4" through (-0.4372, -6.6807, 6) normal (0, 0, -1) x (1, 0, 0)
mirror "Mirror2" about plane through (-0.4372, -6.6807, 6) normal (0, 0, -1) of bodies 2 makes body 7
sketch "Sketch33" plane through (0, 0, 26) normal (0, 0, -1) x (1, 0, 0)
  line L0 (49.5628, 63.1807) -> (-50.4372, 63.1807)
  line L1 (-50.4372, 63.1807) -> (-50.4372, -49.8193)
  line L2 (-50.4372, -49.8193) -> (49.5628, -49.8193)
  line L3 (49.5628, -49.8193) -> (49.5628, 63.1807)
  circle A0 centre (37.5628, 53.1807) radius 5.5
  circle A1 centre (37.5628, 53.1807) radius 2.45
  circle A2 centre (-40.4372, 53.1807) radius 2.45
  circle A3 centre (-40.4372, 53.1807) radius 5.5
  circle A4 centre (-15.1369, -8.1192) radius 5.5
  circle A5 centre (-15.1369, -8.1192) radius 2.45
  dimension "d251" = 4.9
  dimension "d252" = 11
  dimension "d253" = 4.9
  dimension "d254" = 11
  dimension "d255" = 4.9
  dimension "d256" = 11
  dimension "d257" = 80.839
  dimension "d259" = 78
  dimension "d260" = 10
  dimension "d261" = 66.3158
  dimension "d262" = 10
  constraint concentric A0 A1
  constraint concentric A2 A3
  constraint concentric A4 A5
  measures "d251" diameter of A5
  measures "d252" diameter of A4
  measures "d253" diameter of A2
  measures "d254" diameter of A3
  measures "d255" diameter of A1
  measures "d256" diameter of A0
  measures "d257" distance of A0.centre A4.centre
  measures "d259" distance of A0.centre A2.centre
  measures "d260" distance of L0 A0.centre
  measures "d261" distance of A2.centre A4.centre
  measures "d262" distance of L1 A2.centre
extrude "Extrude39" add sketch "Sketch33" along normal up to surface (19 mm away) contours A2 | A5 bodies 2
extrude "Extrude38" add sketch "Sketch33" along normal blind 14.4 contours A2 | A3 | A4 | A5 bodies 2
extrude "Extrude40" add sketch "Sketch33" along normal blind 12 contours A0 | A1 bodies 2
sketch "Sketch34" plane through (0, 0, -14) normal (0, 0, 1) x (-1, 0, 0)
  line L0 (50.4372, 63.1807) -> (-49.5628, 63.1807)
  line L1 (-49.5628, 63.1807) -> (-49.5628, -49.8193)
  line L2 (-49.5628, -49.8193) -> (50.4372, -49.8193)
  line L3 (50.4372, -49.8193) -> (50.4372, 63.1807)
  circle A0 centre (-14.2626, -8.1194) radius 5.5
  circle A1 centre (38.4372, 53.1807) radius 5.5
  circle A2 centre (-39.5628, 53.1807) radius 5.5
  circle A3 centre (-14.2626, -8.1194) radius 2.45
  circle A4 centre (-39.5628, 53.1807) radius 2.45
  circle A5 centre (38.4372, 53.1807) radius 2.45
  dimension "d277" = 80.8392
  dimension "d278" = 78
  dimension "d280" = 11
  dimension "d281" = 4.9
  dimension "d282" = 4.9
  dimension "d283" = 11
  dimension "d284" = 11
  dimension "d285" = 4.9
  dimension "d286" = 10
  dimension "d288" = 10
  dimension "d289" = 66.316
  constraint concentric A0 A3
  constraint concentric A2 A4
  constraint concentric A1 A5
  measures "d277" distance of A1.centre A0.centre
  measures "d278" horizontal distance of A2.centre A1.centre
  measures "d280" diameter of A0
  measures "d281" diameter of A3
  measures "d282" diameter of A5
  measures "d283" diameter of A1
  measures "d284" diameter of A2
  measures "d285" diameter of A4
  measures "d286" distance of L0 A1.centre
  measures "d288" distance of L1 A2.centre
  measures "d289" distance of A0.centre A2.centre
extrude "Extrude43" add sketch "Sketch34" along normal up to surface (19 mm away) contours A3 | A4 | A5 bodies 7
extrude "Extrude44" add sketch "Sketch34" along normal up to surface (16 mm away) contours A0 | A1 | A2 bodies 7
sketch "Sketch35" plane through (53.5628, 0, 0) normal (1, 0, 0) x (0, 1, 0)
  circle A0 centre (35.9784, -8.7066) radius 1.25
  circle A1 centre (31.599, -0.6391) radius 1.25
  circle A2 centre (36.1176, -3.4086) radius 1.25
  circle A3 centre (31.3206, -11.235) radius 1.25
  circle A4 centre (26.9413, -3.1675) radius 1.25
  circle A5 centre (26.8021, -8.4654) radius 1.25
  circle A6 centre (31.4598, -5.937) radius 1.25
  line L0 (-65.1807, 2) -> (-65.1807, -16.5)
  line L1 (-65.1807, -16.5) -> (51.8193, -16.5)
  line L2 (51.8193, -16.5) -> (51.8193, 2)
  line L3 (51.8193, 2) -> (-65.1807, 2)
  line L4 (17.6915, 0.6059) -> (-25.4467, 0.6059) construction
  line L5 (-25.4467, 0.6059) -> (-25.4467, -12.7234) construction
  line L6 (-25.4467, -12.7234) -> (17.6915, -12.7234) construction
  line L7 (17.6915, -12.7234) -> (17.6915, 0.6059) construction
  dimension "d294" = 12
  text T0 "BMO" font "Arial Black" height 12 align right middle in box 43.1383 x 13.3292 at (17.6915, 0.6059) x (-1, 0) y (0, -1) spacing 1 kerned
extrude "Extrude45" cut sketch "Sketch35" against normal blind 1 text T0 bodies 7
ref_plane "WorkPlane5" through (-0.4372, -6.6807, -5) normal (0, 0, -1) x (-1, 0, 0)
mirror "Mirror3" about plane through (-0.4372, -6.6807, -5) normal (0, 0, -1) of bodies 1 makes body 8
sketch "Sketch36" plane through (0, 0, -13) normal (0, 0, -1) x (1, 0, 0)
  line L0 (11.5986, 30.4363) -> (28.0634, 30.4363)
  line L1 (28.0634, 30.4363) -> (20.0901, 16.1809)
  line L2 (20.0901, 16.1809) -> (11.5986, 30.4363)
  arc A0 (36.6796, 36.8191) -> (36.3132, 34) centre (30.5628, 36.1807) ccw
  line L3 (36.6796, 36.8191) -> (40.3994, 36.8191)
  line L4 (40.3994, 36.8191) -> (40.3994, 34)
  line L5 (40.3994, 34) -> (36.3132, 34)
  arc A1 (13.965, 45.3815) -> (14.188, 48) centre (20.0628, 46.1807) ccw
  line L6 (13.965, 45.3815) -> (10, 45.3815)
  line L7 (10, 45.3815) -> (10, 48)
  line L8 (10, 48) -> (14.188, 48)
  line L9 (-13.9372, 19.6807) -> (-27.9372, 19.6807)
  line L10 (-27.9372, 19.6807) -> (-27.9372, 28.6807)
  line L11 (-27.9372, 28.6807) -> (-36.9372, 28.6807)
  line L12 (-36.9372, 28.6807) -> (-36.9372, 42.6807)
  line L13 (-36.9372, 42.6807) -> (-27.9372, 42.6807)
  line L14 (-27.9372, 42.6807) -> (-27.9372, 51.6807)
  line L15 (-27.9372, 51.6807) -> (-13.9372, 51.6807)
  line L16 (-13.9372, 51.6807) -> (-13.9372, 42.6807)
  line L17 (-13.9372, 42.6807) -> (-4.9372, 42.6807)
  line L18 (-4.9372, 42.6807) -> (-4.9372, 28.6807)
  line L19 (-4.9372, 28.6807) -> (-13.9372, 28.6807)
  line L20 (-13.9372, 28.6807) -> (-13.9372, 19.6807)
  line L21 (49.5628, -49.8193) -> (49.5628, 21.1807)
  line L22 (49.5628, 21.1807) -> (52.5628, 21.1807)
  line L23 (52.5628, 21.1807) -> (52.5628, 23.1807)
  line L24 (52.5628, 23.1807) -> (53.5628, 23.1807)
  line L25 (53.5628, 23.1807) -> (53.5628, 34.1807)
  line L26 (53.5628, 34.1807) -> (52.5628, 34.1807)
  line L27 (52.5628, 34.1807) -> (52.5628, 36.1807)
  line L28 (52.5628, 36.1807) -> (49.5628, 36.1807)
  line L29 (49.5628, 36.1807) -> (49.5628, 63.1807)
  line L30 (49.5628, 63.1807) -> (-50.4372, 63.1807)
  line L31 (-50.4372, 63.1807) -> (-50.4372, 28.6807)
  line L32 (-50.4372, 28.6807) -> (-53.4372, 28.6807)
  line L33 (-53.4372, 28.6807) -> (-53.4372, 6.6807)
  line L34 (-53.4372, 6.6807) -> (-50.4372, 6.6807)
  line L35 (-50.4372, 6.6807) -> (-50.4372, -49.8193)
  line L36 (-50.4372, -49.8193) -> (49.5628, -49.8193)
  line L37 (-43.9372, 9.6807) -> (45.0628, 9.6807)
  line L38 (45.0628, 9.6807) -> (45.0628, -48.3193)
  line L39 (45.0628, -48.3193) -> (-43.9372, -48.3193)
  line L40 (-43.9372, -48.3193) -> (-43.9372, 9.6807)
  circle A2 centre (37.7096, 53.8473) radius 6
  circle A3 centre (-38.8729, 53.8473) radius 6
  dimension "d300" = 12
  dimension "d301" = 12
  measures "d300" diameter of A2
  measures "d301" diameter of A3
extrude "Extrude41" add 2 faces at (-10.6832, 8.5142, 11.6) (-35.9835, -52.7858, 11.6) along direction (0, 0, -1) up to surface end surface through (0, 0, 10) normal (0, 0, -1) offset 0 on bodies 2 bodies 2
extrude "Extrude42" add 1 faces at (36.893, -54.3408, 14) along direction (0, 0, -1) up to surface (4 mm away) on bodies 2 bodies 2